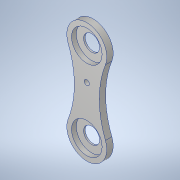
# Autodesk Inventor part: ハンド_リンク1
Saved by Autodesk Inventor 2021 (Build 250183000, 183)
## iProperties
Created: 2021-12-06
Part Number: ハンド_リンク1
Material: アルミニウム 6061
Document SubType Name: Modeling
Designer: 堀川皓史
Density: 2.7 g/cm^3
Appearance: アルミニウム - フラット
Mass: 10.9488 g
Surface Area: 37.4873 cm^2
Volume: 4.05512 cm^3
Author: 堀川皓史
Autodesk Inventor part; units mm, degrees
ref_plane "YZ Plane" through (0, 0, 0) normal (1, 0, 0) x (0, 1, 0)
ref_plane "XZ Plane" through (0, 0, 0) normal (0, 1, 0) x (-1, 0, 0)
ref_plane "XY Plane" through (0, 0, 0) normal (0, 0, 1) x (1, 0, 0)
sketch "スケッチ1" plane through (0, 0, 0) normal (0, 0, 1) x (1, 0, 0)
  circle A0 centre (0, 0) radius 5
  circle A1 centre (0, 50) radius 5
  arc A2 (11.6485, 45.4655) -> (-11.6485, 45.4655) centre (0, 50) ccw
  arc A3 (-11.6485, 4.5345) -> (11.6485, 4.5345) centre (0, 0) ccw
  circle A4 centre (0, 30) radius 1.6
  circle A5 centre (0, 30) radius 8 construction
  arc A6 (-11.6485, 4.5345) -> (-11.6485, 45.4655) centre (-64.2223, 25) ccw
  arc A7 (11.6485, 45.4655) -> (11.6485, 4.5345) centre (64.2223, 25) ccw
  dimension "d0" = 10
  dimension "d1" = 10
  dimension "d2" = 50
  dimension "d3" = 12.5
  dimension "d4" = 12.5
  dimension "d11" = 3.2
  dimension "d12" = 20
  dimension "d13" = 16
  constraints: 8 centre point, 8 point on circle, 6 tangent, 4 coincident, 2 vertical alignment
  measures "d0" diameter of A0
  measures "d1" diameter of A1
  measures "d2" distance of point (0, 0) A1.centre
  measures "d3" radius of A2
  measures "d4" radius of A3
  measures "d11" diameter of A4
  measures "d12" distance of A4.centre A1.centre
  measures "d13" diameter of A5
extrude "押し出し1" add sketch "スケッチ1" along normal blind 4
sketch "スケッチ2" plane through (0, 0, 4) normal (0, 0, 1) x (1, 0, 0)
  circle A0 centre (0, 0) radius 9.55
  circle A1 centre (0, 50) radius 5 projected
  circle A2 centre (0, 50) radius 9.55
  dimension "d7" = 19.1
  dimension "d8" = 19.1
  constraints: 2 centre point, 2 coincident
  measures "d7" diameter of A0
  measures "d8" diameter of A2
extrude "押し出し2" cut sketch "スケッチ2" against normal blind 3
